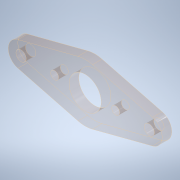
# Autodesk Inventor part: エンコーダマウント
Saved by Autodesk Inventor 2021 (Build 250183000, 183)
## iProperties
Created: 2022-02-01
Part Number: エンコーダマウント
Material: ポリカーボネート、スモーク
Document SubType Name: Modeling
Designer: hirohumi
Density: 1.2 g/cm^3
Appearance: ポリカーボネート - スモーク
Author: hirohumi
Autodesk Inventor part; units mm, degrees
ref_plane "YZ Plane" through (0, 0, 0) normal (1, 0, 0) x (0, 1, 0)
ref_plane "XZ Plane" through (0, 0, 0) normal (0, 1, 0) x (-1, 0, 0)
ref_plane "XY Plane" through (0, 0, 0) normal (0, 0, 1) x (1, 0, 0)
sketch "スケッチ1" plane through (0, 0, 0) normal (0, 0, 1) x (1, 0, 0)
  circle A0 centre (0, 0) radius 5
  circle A1 centre (-20, 0) radius 1.6
  circle A2 centre (20, 0) radius 1.6
  circle A3 centre (-9.525, 0) radius 1.25
  circle A4 centre (9.525, 0) radius 1.25
  line L0 (-20, 0) -> (20, 0) construction
  arc A5 (-21, 3.873) -> (-21, -3.873) centre (-20, 0) ccw
  arc A6 (21, -3.873) -> (21, 3.873) centre (20, 0) ccw
  arc A7 (2.25, 8.7142) -> (-2.25, 8.7142) centre (0, 0) ccw
  arc A8 (-2.25, -8.7142) -> (2.25, -8.7142) centre (0, 0) ccw
  line L1 (-21, 3.873) -> (-2.25, 8.7142)
  line L2 (2.25, 8.7142) -> (21, 3.873)
  line L3 (21, -3.873) -> (2.25, -8.7142)
  line L4 (-2.25, -8.7142) -> (-21, -3.873)
  dimension "d0" = 10
  dimension "d1" = 3.2
  dimension "d2" = 3.2
  dimension "d3" = 40
  dimension "d4" = 20
  dimension "d5" = 2.5
  dimension "d6" = 2.5
  dimension "d7" = 19.05
  dimension "d8" = 9.525
  dimension "d9" = 4
  dimension "d10" = 4
  dimension "d11" = 9
  dimension "d12" = 9
  constraints: 10 end point, 9 centre point, 8 point on circle, 8 tangent, 5 coincident, 2 horizontal alignment, 2 point on line, 1 horizontal
  measures "d0" diameter of A0
  measures "d1" diameter of A1
  measures "d2" diameter of A2
  measures "d3" distance of L0.end L0.start
  measures "d4" distance of point (0, 0) L0.start
  measures "d5" diameter of A3
  measures "d6" diameter of A4
  measures "d7" distance of A4.centre A3.centre
  measures "d8" distance of point (0, 0) A3.centre
  measures "d9" radius of A5
  measures "d10" radius of A6
  measures "d11" radius of A7
  measures "d12" radius of A8
extrude "押し出し1" add sketch "スケッチ1" along normal blind 3
equation "\"d8\" = 0.5 * d7"
